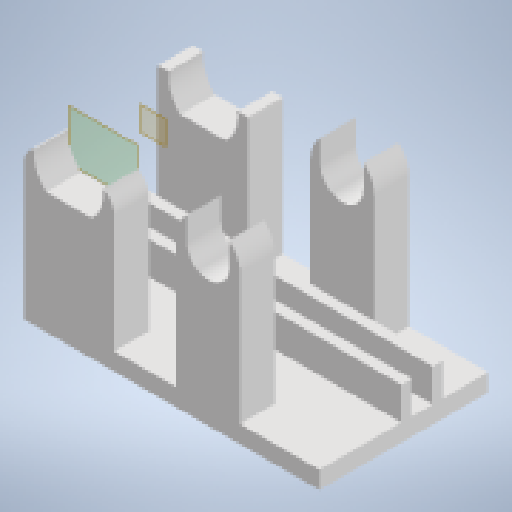
# Autodesk Inventor part: tempMotorHolder_V3
Saved by Autodesk Inventor 2023 (Build 270158000, 158)
## iProperties
Created: 2022-11-25
Part Number: tempMotorHolder_V3
Material: Generic
Document SubType Name: Modeling
Designer: shrey
Density: 1 g/cm^3
Appearance: Default
Author: shrey
Autodesk Inventor part; units mm, degrees
(part 1 of 2)
ref_plane "YZ Plane" through (0, 0, 0) normal (1, 0, 0) x (0, 1, 0)
ref_plane "XZ Plane" through (0, 0, 0) normal (0, 1, 0) x (-1, 0, 0)
ref_plane "XY Plane" through (0, 0, 0) normal (0, 0, 1) x (1, 0, 0)
ref_plane "Work Plane1" through (24.9677, 22.5561, 7.78) normal (0, 0, 1) x (1, 0, 0)
ref_plane "Work Plane2" through (24.8534, 22.5561, 22.06) normal (0, 0, -1) x (-1, 0, 0)
sketch "Sketch1" plane through (24.8534, 22.5561, 22.06) normal (0, 0, -1) x (-1, 0, 0)
  line L0 (6.3856, -7.5) -> (-6.6144, -7.5) construction
  line L1 (-6.6144, 7.5) -> (6.3856, 7.5) construction
  arc A0 (6.3856, -7.5) -> (6.3856, 7.5) centre (-0.2288, 0) ccw construction
  arc A1 (-6.6144, 7.5) -> (-6.6144, -7.5) centre (0, 0) ccw construction
  line L2 (6.4233, 7.6) -> (-6.6521, 7.6)
  arc A2 (-6.6521, 7.6) -> (-6.6521, -7.6) centre (0, 0) ccw
  line L3 (-6.6521, -7.6) -> (6.4233, -7.6)
  arc A3 (6.4233, -7.6) -> (6.4233, 7.6) centre (-0.2288, 0) ccw
  line L4 (9.7712, 0) -> (9.7712, 14.6932)
  line L5 (-10, 0) -> (-10, 14.6932)
  spline S0 degree 3 poles (-32.7358, 31.1377) (-32.7075, 31.029) (-32.6509, 30.8115) (-32.5759, 30.4828) (-32.5083, 30.1525) (-32.4494, 29.8206) (-32.3995, 29.4872) (-32.3592, 29.1525) (-32.3295, 28.8167) (-32.3114, 28.4801) (-32.307, 28.1991) (-32.3108, 27.9744) (-32.3179, 27.806) (-32.3291, 27.6378) (-32.3467, 27.4702) (-32.3629, 27.3307) (-32.3682, 27.2184) (-32.3676, 27.1341) (-32.3634, 27.0499) (-32.3544, 26.9661) (-32.3399, 26.883) (-32.3196, 26.8011) (-32.2931, 26.7211) (-32.2601, 26.6434) (-32.2203, 26.569) (-32.1734, 26.4988) (-32.12, 26.4335) (-32.0614, 26.3729) (-31.9958, 26.3197) (-31.9255, 26.2731) (-31.851, 26.2334) (-31.7455, 26.1941) (-31.611, 26.1536) (-31.4784, 26.1073) (-31.3701, 26.077) (-31.2864, 26.0653) (-31.2022, 26.0616) (-31.1178, 26.0661) (-31.0347, 26.0807) (-30.9532, 26.1021) (-30.874, 26.1312) (-30.798, 26.1681) (-30.7257, 26.2114) (-30.6571, 26.2606) (-30.5926, 26.3148) (-30.532, 26.3735) (-30.4754, 26.436) (-30.4225, 26.5017) (-30.3724, 26.5695) (-30.3107, 26.6634) (-30.2417, 26.7858) (-30.1574, 26.9317) (-30.0676, 27.0744) (-29.9742, 27.2147) (-29.8452, 27.3987) (-29.6764, 27.6233) (-29.4638, 27.8849) (-29.2422, 28.1391) (-29.0129, 28.3861) (-28.7764, 28.6264) (-28.5336, 28.8602) (-28.2847, 29.0876) (-28.0307, 29.3093) (-27.8571, 29.4519) (-27.7702, 29.5232) knots -1.078574 -1.078574 -1.078574 -1.078574 -1.044867 -1.011159 -0.977452 -0.943745 -0.910038 -0.876331 -0.842624 -0.808918 -0.775212 -0.758359 -0.741505 -0.724651 -0.707798 -0.690947 -0.68252 -0.674093 -0.665668 -0.657242 -0.648815 -0.640389 -0.631963 -0.623537 -0.61511 -0.606685 -0.598264 -0.589839 -0.581413 -0.57299 -0.564565 -0.556141 -0.539287 -0.522433 -0.514009 -0.505584 -0.49716 -0.488735 -0.48031 -0.471889 -0.463464 -0.455037 -0.446611 -0.438185 -0.429758 -0.421332 -0.412906 -0.40448 -0.396053 -0.387627 -0.370775 -0.353922 -0.337069 -0.320215 -0.303361 -0.269656 -0.235949 -0.202243 -0.168536 -0.134829 -0.101122 -0.067415 -0.033707 0 0 0 0 construction
  arc A4 (-26.4231, 28.9232) -> (-27.7702, 29.5232) centre (-40.1144, 0) ccw construction
  spline S1 degree 3 poles (-26.4231, 28.9232) (-26.4181, 28.8109) (-26.408, 28.5864) (-26.4029, 28.2493) (-26.4055, 27.9122) (-26.4168, 27.5753) (-26.4373, 27.2388) (-26.4676, 26.9031) (-26.5083, 26.5684) (-26.5606, 26.2354) (-26.6146, 25.9596) (-26.6651, 25.7407) (-26.707, 25.5774) (-26.753, 25.4152) (-26.8051, 25.2549) (-26.8499, 25.1218) (-26.8785, 25.0131) (-26.8954, 24.9305) (-26.9088, 24.8473) (-26.9174, 24.7634) (-26.9206, 24.6791) (-26.9177, 24.5948) (-26.9084, 24.511) (-26.8922, 24.4282) (-26.8688, 24.3471) (-26.8375, 24.2688) (-26.7989, 24.1938) (-26.7541, 24.1222) (-26.7011, 24.0566) (-26.642, 23.9964) (-26.5773, 23.9421) (-26.4823, 23.8817) (-26.3592, 23.8141) (-26.2391, 23.7413) (-26.1394, 23.6891) (-26.0601, 23.6603) (-25.9784, 23.6392) (-25.895, 23.626) (-25.8107, 23.623) (-25.7264, 23.627) (-25.6429, 23.639) (-25.561, 23.6592) (-25.4812, 23.6866) (-25.4039, 23.7204) (-25.3295, 23.7601) (-25.258, 23.8049) (-25.1897, 23.8543) (-25.1243, 23.9075) (-25.0612, 23.9634) (-24.9813, 24.0425) (-24.8884, 24.1479) (-24.7756, 24.2731) (-24.658, 24.3939) (-24.5376, 24.5118) (-24.3731, 24.6649) (-24.1613, 24.8495) (-23.8989, 25.0612) (-23.6294, 25.2637) (-23.3537, 25.4577) (-23.0724, 25.6436) (-22.7863, 25.8218) (-22.4955, 25.9924) (-22.201, 26.1565) (-22.0015, 26.2599) (-21.9018, 26.3116) knots -1.078574 -1.078574 -1.078574 -1.078574 -1.044867 -1.011159 -0.977452 -0.943745 -0.910038 -0.876331 -0.842624 -0.808918 -0.775212 -0.758359 -0.741505 -0.724651 -0.707798 -0.690947 -0.68252 -0.674093 -0.665668 -0.657242 -0.648815 -0.640389 -0.631963 -0.623537 -0.61511 -0.606685 -0.598264 -0.589839 -0.581413 -0.57299 -0.564565 -0.556141 -0.539287 -0.522433 -0.514009 -0.505584 -0.49716 -0.488735 -0.48031 -0.471889 -0.463464 -0.455037 -0.446611 -0.438185 -0.429758 -0.421332 -0.412906 -0.40448 -0.396053 -0.387627 -0.370775 -0.353922 -0.337069 -0.320215 -0.303361 -0.269656 -0.235949 -0.202243 -0.168536 -0.134829 -0.101122 -0.067415 -0.033707 0 0 0 0 construction
  arc A5 (-20.7088, 25.4446) -> (-21.9018, 26.3116) centre (-40.1144, 0) ccw construction
  spline S2 degree 3 poles (-20.7088, 25.4446) (-20.7272, 25.3337) (-20.764, 25.112) (-20.8292, 24.7812) (-20.9017, 24.4521) (-20.9829, 24.1249) (-21.0729, 23.8) (-21.1723, 23.4778) (-21.2818, 23.159) (-21.4021, 22.8441) (-21.5123, 22.5856) (-21.6073, 22.3819) (-21.6822, 22.2309) (-21.7608, 22.0818) (-21.8451, 21.9359) (-21.9167, 21.815) (-21.9672, 21.7146) (-22.0009, 21.6373) (-22.0313, 21.5587) (-22.0572, 21.4785) (-22.0778, 21.3967) (-22.0925, 21.3136) (-22.1008, 21.2297) (-22.1023, 21.1453) (-22.0962, 21.0612) (-22.0819, 20.978) (-22.0597, 20.8967) (-22.0308, 20.8174) (-21.9925, 20.7421) (-21.9472, 20.6709) (-21.8953, 20.6043) (-21.8149, 20.5256) (-21.7086, 20.4339) (-21.6063, 20.3377) (-21.5196, 20.2659) (-21.4479, 20.2212) (-21.3724, 20.1836) (-21.2936, 20.1533) (-21.2117, 20.1328) (-21.1285, 20.1193) (-21.0443, 20.1136) (-20.96, 20.1164) (-20.8762, 20.1266) (-20.7936, 20.1436) (-20.7125, 20.1669) (-20.6334, 20.1959) (-20.5562, 20.23) (-20.4812, 20.2685) (-20.4079, 20.31) (-20.3133, 20.3707) (-20.2005, 20.4545) (-20.0641, 20.5535) (-19.924, 20.6473) (-19.7817, 20.7375) (-19.589, 20.8531) (-19.3434, 20.9897) (-19.0427, 21.1422) (-18.737, 21.2842) (-18.427, 21.4166) (-18.1132, 21.54) (-17.7963, 21.6548) (-17.4764, 21.7613) (-17.1542, 21.8605) (-16.9376, 21.9202) (-16.8293, 21.95) knots -1.078574 -1.078574 -1.078574 -1.078574 -1.044867 -1.011159 -0.977452 -0.943745 -0.910038 -0.876331 -0.842624 -0.808918 -0.775212 -0.758359 -0.741505 -0.724651 -0.707798 -0.690947 -0.68252 -0.674093 -0.665668 -0.657242 -0.648815 -0.640389 -0.631963 -0.623537 -0.61511 -0.606685 -0.598264 -0.589839 -0.581413 -0.57299 -0.564565 -0.556141 -0.539287 -0.522433 -0.514009 -0.505584 -0.49716 -0.488735 -0.48031 -0.471889 -0.463464 -0.455037 -0.446611 -0.438185 -0.429758 -0.421332 -0.412906 -0.40448 -0.396053 -0.387627 -0.370775 -0.353922 -0.337069 -0.320215 -0.303361 -0.269656 -0.235949 -0.202243 -0.168536 -0.134829 -0.101122 -0.067415 -0.033707 0 0 0 0 construction
  arc A6 (-15.8427, 20.8539) -> (-16.8293, 21.95) centre (-40.1144, 0) ccw construction
  spline S3 degree 3 poles (-15.8427, 20.8539) (-15.8837, 20.7493) (-15.9658, 20.5401) (-16.0983, 20.2301) (-16.2377, 19.9232) (-16.3851, 19.62) (-16.5407, 19.3209) (-16.7049, 19.0265) (-16.8783, 18.7374) (-17.0615, 18.4544) (-17.223, 18.2245) (-17.3582, 18.045) (-17.4629, 17.9129) (-17.5708, 17.7834) (-17.6836, 17.6581) (-17.7787, 17.5548) (-17.8491, 17.4671) (-17.8981, 17.3985) (-17.9442, 17.3279) (-17.9862, 17.2548) (-18.0233, 17.1791) (-18.055, 17.1009) (-18.0806, 17.0205) (-18.0995, 16.9383) (-18.1111, 16.8547) (-18.1144, 16.7704) (-18.1096, 16.6862) (-18.0978, 16.6027) (-18.076, 16.5211) (-18.0465, 16.4421) (-18.0095, 16.3661) (-17.9473, 16.2724) (-17.8624, 16.1605) (-17.7823, 16.0452) (-17.7124, 15.957) (-17.6516, 15.8983) (-17.5856, 15.8458) (-17.5148, 15.7999) (-17.4389, 15.7628) (-17.3604, 15.7322) (-17.2792, 15.7092) (-17.1961, 15.6944) (-17.1121, 15.687) (-17.0277, 15.6864) (-16.9436, 15.6924) (-16.8601, 15.7042) (-16.7776, 15.7216) (-16.6962, 15.7436) (-16.6158, 15.769) (-16.5107, 15.8087) (-16.3829, 15.8672) (-16.2289, 15.9357) (-16.0724, 15.9983) (-15.9144, 16.0569) (-15.7019, 16.13) (-15.4333, 16.2125) (-15.1075, 16.2991) (-14.7789, 16.3745) (-14.4481, 16.4396) (-14.1156, 16.495) (-13.7817, 16.5414) (-13.4467, 16.579) (-13.1109, 16.6091) (-12.8866, 16.6224) (-12.7744, 16.6291) knots -1.078574 -1.078574 -1.078574 -1.078574 -1.044867 -1.011159 -0.977452 -0.943745 -0.910038 -0.876331 -0.842624 -0.808918 -0.775212 -0.758359 -0.741505 -0.724651 -0.707798 -0.690947 -0.68252 -0.674093 -0.665668 -0.657242 -0.648815 -0.640389 -0.631963 -0.623537 -0.61511 -0.606685 -0.598264 -0.589839 -0.581413 -0.57299 -0.564565 -0.556141 -0.539287 -0.522433 -0.514009 -0.505584 -0.49716 -0.488735 -0.48031 -0.471889 -0.463464 -0.455037 -0.446611 -0.438185 -0.429758 -0.421332 -0.412906 -0.40448 -0.396053 -0.387627 -0.370775 -0.353922 -0.337069 -0.320215 -0.303361 -0.269656 -0.235949 -0.202243 -0.168536 -0.134829 -0.101122 -0.067415 -0.033707 0 0 0 0 construction
  arc A7 (-12.0373, 15.3518) -> (-12.7744, 16.6291) centre (-40.1144, 0) ccw construction
  spline S4 degree 3 poles (-12.0373, 15.3518) (-12.0992, 15.258) (-12.223, 15.0705) (-12.417, 14.7948) (-12.6172, 14.5236) (-12.8245, 14.2577) (-13.0388, 13.9975) (-13.2606, 13.7437) (-13.4903, 13.4969) (-13.7283, 13.2581) (-13.9342, 13.0668) (-14.1037, 12.9194) (-14.2336, 12.8119) (-14.3661, 12.7077) (-14.5024, 12.6086) (-14.617, 12.5273) (-14.704, 12.4561) (-14.7662, 12.3993) (-14.826, 12.3398) (-14.8823, 12.277) (-14.9343, 12.2107) (-14.9816, 12.1408) (-15.0233, 12.0675) (-15.0589, 11.991) (-15.0876, 11.9117) (-15.1083, 11.8299) (-15.1212, 11.7465) (-15.127, 11.6624) (-15.1227, 11.578) (-15.1102, 11.4946) (-15.0899, 11.4126) (-15.0485, 11.308) (-14.9887, 11.1809) (-14.9343, 11.0514) (-14.8843, 10.9506) (-14.837, 10.8806) (-14.7834, 10.8156) (-14.7236, 10.7559) (-14.6572, 10.7039) (-14.5867, 10.6576) (-14.512, 10.6182) (-14.4339, 10.5864) (-14.3532, 10.5617) (-14.2708, 10.5436) (-14.1873, 10.532) (-14.1032, 10.5262) (-14.0188, 10.526) (-13.9347, 10.5306) (-13.8508, 10.5388) (-13.7397, 10.5558) (-13.6025, 10.5864) (-13.4377, 10.6214) (-13.2716, 10.6501) (-13.1048, 10.6746) (-12.8817, 10.7018) (-12.6019, 10.7267) (-12.2652, 10.7437) (-11.9281, 10.7491) (-11.591, 10.744) (-11.2542, 10.7291) (-10.918, 10.705) (-10.5825, 10.6722) (-10.2478, 10.6318) (-10.0256, 10.5982) (-9.9145, 10.5814) knots -1.078574 -1.078574 -1.078574 -1.078574 -1.044867 -1.011159 -0.977452 -0.943745 -0.910038 -0.876331 -0.842624 -0.808918 -0.775212 -0.758359 -0.741505 -0.724651 -0.707798 -0.690947 -0.68252 -0.674093 -0.665668 -0.657242 -0.648815 -0.640389 -0.631963 -0.623537 -0.61511 -0.606685 -0.598264 -0.589839 -0.581413 -0.57299 -0.564565 -0.556141 -0.539287 -0.522433 -0.514009 -0.505584 -0.49716 -0.488735 -0.48031 -0.471889 -0.463464 -0.455037 -0.446611 -0.438185 -0.429758 -0.421332 -0.412906 -0.40448 -0.396053 -0.387627 -0.370775 -0.353922 -0.337069 -0.320215 -0.303361 -0.269656 -0.235949 -0.202243 -0.168536 -0.134829 -0.101122 -0.067415 -0.033707 0 0 0 0 construction
  arc A8 (-9.459, 9.1788) -> (-9.9145, 10.5814) centre (-40.1144, 0) ccw construction
  spline S5 degree 3 poles (-9.459, 9.1788) (-9.5391, 9.0999) (-9.6991, 8.9422) (-9.9463, 8.7129) (-10.1985, 8.4892) (-10.4565, 8.2722) (-10.7202, 8.0623) (-10.99, 7.8601) (-11.266, 7.6665) (-11.5484, 7.4824) (-11.7895, 7.3381) (-11.986, 7.2291) (-12.1354, 7.151) (-12.2867, 7.0766) (-12.4406, 7.0081) (-12.5696, 6.9523) (-12.6695, 6.9008) (-12.7422, 6.8581) (-12.813, 6.8124) (-12.8811, 6.7627) (-12.9458, 6.7086) (-13.0066, 6.6501) (-13.0626, 6.5871) (-13.1134, 6.5197) (-13.158, 6.448) (-13.1952, 6.3723) (-13.2251, 6.2935) (-13.2483, 6.2123) (-13.2616, 6.129) (-13.2668, 6.0448) (-13.2639, 5.9604) (-13.2451, 5.8494) (-13.2131, 5.7127) (-13.1868, 5.5747) (-13.1589, 5.4657) (-13.1272, 5.3874) (-13.0882, 5.3126) (-13.0422, 5.2418) (-12.988, 5.1771) (-12.9287, 5.1172) (-12.8639, 5.0632) (-12.794, 5.0158) (-12.7203, 4.9749) (-12.6434, 4.9401) (-12.5641, 4.9113) (-12.483, 4.8882) (-12.4006, 4.8704) (-12.3173, 4.8574) (-12.2336, 4.848) (-12.1213, 4.8415) (-11.9809, 4.843) (-11.8123, 4.8429) (-11.6439, 4.8364) (-11.4757, 4.8257) (-11.2518, 4.806) (-10.9729, 4.7721) (-10.64, 4.7188) (-10.3092, 4.654) (-9.9805, 4.5789) (-9.6542, 4.4943) (-9.3303, 4.4008) (-9.0089, 4.299) (-8.69, 4.1899) (-8.4796, 4.1108) (-8.3744, 4.0713) knots -1.078574 -1.078574 -1.078574 -1.078574 -1.044867 -1.011159 -0.977452 -0.943745 -0.910038 -0.876331 -0.842624 -0.808918 -0.775212 -0.758359 -0.741505 -0.724651 -0.707798 -0.690947 -0.68252 -0.674093 -0.665668 -0.657242 -0.648815 -0.640389 -0.631963 -0.623537 -0.61511 -0.606685 -0.598264 -0.589839 -0.581413 -0.57299 -0.564565 -0.556141 -0.539287 -0.522433 -0.514009 -0.505584 -0.49716 -0.488735 -0.48031 -0.471889 -0.463464 -0.455037 -0.446611 -0.438185 -0.429758 -0.421332 -0.412906 -0.40448 -0.396053 -0.387627 -0.370775 -0.353922 -0.337069 -0.320215 -0.303361 -0.269656 -0.235949 -0.202243 -0.168536 -0.134829 -0.101122 -0.067415 -0.033707 0 0 0 0 construction
  arc A9 (-8.2206, 2.6046) -> (-8.3744, 4.0713) centre (-40.1144, 0) ccw construction
  spline S6 degree 3 poles (-8.2206, 2.6046) (-8.3152, 2.5441) (-8.5046, 2.4231) (-8.794, 2.2502) (-9.0872, 2.0839) (-9.3847, 1.9252) (-9.6863, 1.7747) (-9.9922, 1.6331) (-10.3024, 1.501) (-10.617, 1.3797) (-10.8828, 1.2887) (-11.0977, 1.2229) (-11.26, 1.1776) (-11.4235, 1.1363) (-11.5883, 1.1013) (-11.726, 1.0735) (-11.8345, 1.0439) (-11.9144, 1.0173) (-11.9932, 0.9873) (-12.0702, 0.9528) (-12.1447, 0.9134) (-12.2163, 0.8688) (-12.2842, 0.8188) (-12.3479, 0.7634) (-12.4064, 0.7026) (-12.4586, 0.6363) (-12.5042, 0.5653) (-12.5438, 0.4908) (-12.5741, 0.412) (-12.5967, 0.3307) (-12.6114, 0.2476) (-12.6161, 0.1352) (-12.6132, -0.0053) (-12.6162, -0.1457) (-12.6115, -0.2581) (-12.5968, -0.3413) (-12.5743, -0.4225) (-12.544, -0.5014) (-12.5044, -0.5759) (-12.4588, -0.6468) (-12.4067, -0.7132) (-12.3482, -0.774) (-12.2846, -0.8294) (-12.2166, -0.8794) (-12.1451, -0.9241) (-12.0705, -0.9635) (-11.9936, -0.998) (-11.9148, -1.028) (-11.8349, -1.0547) (-11.7265, -1.0844) (-11.5887, -1.1122) (-11.4239, -1.1473) (-11.2605, -1.1886) (-11.0982, -1.234) (-10.8833, -1.2999) (-10.6175, -1.391) (-10.303, -1.5124) (-9.9929, -1.6446) (-9.687, -1.7864) (-9.3854, -1.937) (-9.088, -2.0957) (-8.7949, -2.2622) (-8.5055, -2.4352) (-8.3162, -2.5563) (-8.2216, -2.6168) knots -1.078574 -1.078574 -1.078574 -1.078574 -1.044867 -1.011159 -0.977452 -0.943745 -0.910038 -0.876331 -0.842624 -0.808918 -0.775212 -0.758359 -0.741505 -0.724651 -0.707798 -0.690947 -0.68252 -0.674093 -0.665668 -0.657242 -0.648815 -0.640389 -0.631963 -0.623537 -0.61511 -0.606685 -0.598264 -0.589839 -0.581413 -0.57299 -0.564565 -0.556141 -0.539287 -0.522433 -0.514009 -0.505584 -0.49716 -0.488735 -0.48031 -0.471889 -0.463464 -0.455037 -0.446611 -0.438185 -0.429758 -0.421332 -0.412906 -0.40448 -0.396053 -0.387627 -0.370775 -0.353922 -0.337069 -0.320215 -0.303361 -0.269656 -0.235949 -0.202243 -0.168536 -0.134829 -0.101122 -0.067415 -0.033707 0 0 0 0 construction
  arc A10 (-8.376, -4.0834) -> (-8.2216, -2.6168) centre (-40.1144, 0) ccw construction
  spline S7 degree 3 poles (-8.376, -4.0834) (-8.4812, -4.1229) (-8.6916, -4.2019) (-9.0106, -4.3109) (-9.332, -4.4126) (-9.6559, -4.5059) (-9.9823, -4.5904) (-10.3109, -4.6654) (-10.6418, -4.73) (-10.9747, -4.7833) (-11.2536, -4.817) (-11.4775, -4.8367) (-11.6457, -4.8473) (-11.8142, -4.8537) (-11.9827, -4.8537) (-12.1232, -4.8522) (-12.2354, -4.8586) (-12.3192, -4.8681) (-12.4025, -4.881) (-12.4849, -4.8987) (-12.566, -4.9218) (-12.6453, -4.9506) (-12.7222, -4.9853) (-12.7959, -5.0263) (-12.8658, -5.0736) (-12.9306, -5.1276) (-12.99, -5.1875) (-13.0442, -5.2522) (-13.0903, -5.3229) (-13.1292, -5.3977) (-13.1609, -5.476) (-13.1889, -5.585) (-13.2152, -5.723) (-13.2474, -5.8597) (-13.2662, -5.9706) (-13.2691, -6.055) (-13.2639, -6.1392) (-13.2507, -6.2226) (-13.2275, -6.3037) (-13.1977, -6.3826) (-13.1604, -6.4584) (-13.1159, -6.53) (-13.0651, -6.5974) (-13.0091, -6.6605) (-12.9484, -6.719) (-12.8837, -6.7731) (-12.8156, -6.8228) (-12.7448, -6.8686) (-12.6722, -6.9113) (-12.5723, -6.9629) (-12.4433, -7.0187) (-12.2894, -7.0873) (-12.1381, -7.1617) (-11.9888, -7.2399) (-11.7923, -7.349) (-11.5513, -7.4933) (-11.2689, -7.6775) (-10.993, -7.8712) (-10.7233, -8.0735) (-10.4596, -8.2836) (-10.2017, -8.5007) (-9.9496, -8.7244) (-9.7026, -8.9538) (-9.5426, -9.1116) (-9.4625, -9.1905) knots -1.078574 -1.078574 -1.078574 -1.078574 -1.044867 -1.011159 -0.977452 -0.943745 -0.910038 -0.876331 -0.842624 -0.808918 -0.775212 -0.758359 -0.741505 -0.724651 -0.707798 -0.690947 -0.68252 -0.674093 -0.665668 -0.657242 -0.648815 -0.640389 -0.631963 -0.623537 -0.61511 -0.606685 -0.598264 -0.589839 -0.581413 -0.57299 -0.564565 -0.556141 -0.539287 -0.522433 -0.514009 -0.505584 -0.49716 -0.488735 -0.48031 -0.471889 -0.463464 -0.455037 -0.446611 -0.438185 -0.429758 -0.421332 -0.412906 -0.40448 -0.396053 -0.387627 -0.370775 -0.353922 -0.337069 -0.320215 -0.303361 -0.269656 -0.235949 -0.202243 -0.168536 -0.134829 -0.101122 -0.067415 -0.033707 0 0 0 0 construction
  arc A11 (-9.9185, -10.593) -> (-9.4625, -9.1905) centre (-40.1144, 0) ccw construction
  spline S8 degree 3 poles (-9.9185, -10.593) (-10.0296, -10.6097) (-10.2518, -10.6432) (-10.5866, -10.6835) (-10.9221, -10.7162) (-11.2583, -10.7401) (-11.5951, -10.7549) (-11.9322, -10.7599) (-12.2693, -10.7543) (-12.606, -10.7372) (-12.8858, -10.7123) (-13.1089, -10.6849) (-13.2756, -10.6603) (-13.4417, -10.6316) (-13.6066, -10.5966) (-13.7437, -10.5659) (-13.8548, -10.5488) (-13.9387, -10.5406) (-14.0229, -10.536) (-14.1072, -10.5362) (-14.1913, -10.5419) (-14.2749, -10.5535) (-14.3573, -10.5716) (-14.4379, -10.5963) (-14.5161, -10.628) (-14.5908, -10.6674) (-14.6613, -10.7136) (-14.7278, -10.7656) (-14.7875, -10.8252) (-14.8412, -10.8903) (-14.8885, -10.9603) (-14.9385, -11.0611) (-14.9929, -11.1905) (-15.0528, -11.3176) (-15.0942, -11.4222) (-15.1146, -11.5042) (-15.1271, -11.5876) (-15.1315, -11.6719) (-15.1257, -11.7561) (-15.1129, -11.8394) (-15.0922, -11.9213) (-15.0635, -12.0006) (-15.0279, -12.0771) (-14.9862, -12.1504) (-14.939, -12.2203) (-14.887, -12.2867) (-14.8307, -12.3495) (-14.771, -12.4089) (-14.7088, -12.4658) (-14.6218, -12.537) (-14.5073, -12.6184) (-14.371, -12.7175) (-14.2385, -12.8218) (-14.1087, -12.9293) (-13.9392, -13.0769) (-13.7334, -13.2682) (-13.4955, -13.5071) (-13.2659, -13.7539) (-13.0442, -14.0078) (-12.8299, -14.2681) (-12.6228, -14.5341) (-12.4227, -14.8054) (-12.2287, -15.0811) (-12.105, -15.2687) (-12.0432, -15.3625) knots -1.078574 -1.078574 -1.078574 -1.078574 -1.044867 -1.011159 -0.977452 -0.943745 -0.910038 -0.876331 -0.842624 -0.808918 -0.775212 -0.758359 -0.741505 -0.724651 -0.707798 -0.690947 -0.68252 -0.674093 -0.665668 -0.657242 -0.648815 -0.640389 -0.631963 -0.623537 -0.61511 -0.606685 -0.598264 -0.589839 -0.581413 -0.57299 -0.564565 -0.556141 -0.539287 -0.522433 -0.514009 -0.505584 -0.49716 -0.488735 -0.48031 -0.471889 -0.463464 -0.455037 -0.446611 -0.438185 -0.429758 -0.421332 -0.412906 -0.40448 -0.396053 -0.387627 -0.370775 -0.353922 -0.337069 -0.320215 -0.303361 -0.269656 -0.235949 -0.202243 -0.168536 -0.134829 -0.101122 -0.067415 -0.033707 0 0 0 0 construction
  arc A12 (-12.7808, -16.6395) -> (-12.0432, -15.3625) centre (-40.1144, 0) ccw construction
  spline S9 degree 3 poles (-12.7808, -16.6395) (-12.8929, -16.6328) (-13.1173, -16.6194) (-13.453, -16.5892) (-13.788, -16.5514) (-14.1219, -16.5049) (-14.4544, -16.4494) (-14.7852, -16.3842) (-15.1137, -16.3087) (-15.4395, -16.2219) (-15.7081, -16.1393) (-15.9206, -16.0662) (-16.0785, -16.0075) (-16.235, -15.9448) (-16.389, -15.8763) (-16.5167, -15.8177) (-16.6219, -15.778) (-16.7022, -15.7525) (-16.7836, -15.7305) (-16.8661, -15.7131) (-16.9496, -15.7012) (-17.0337, -15.6952) (-17.1181, -15.6957) (-17.2021, -15.7031) (-17.2852, -15.7179) (-17.3664, -15.7409) (-17.445, -15.7715) (-17.5208, -15.8085) (-17.5917, -15.8544) (-17.6577, -15.9069) (-17.7185, -15.9655) (-17.7884, -16.0537) (-17.8685, -16.169) (-17.9535, -16.2809) (-18.0158, -16.3746) (-18.0528, -16.4505) (-18.0823, -16.5295) (-18.1041, -16.6111) (-18.116, -16.6946) (-18.1208, -16.7788) (-18.1176, -16.8632) (-18.106, -16.9467) (-18.0871, -17.029) (-18.0615, -17.1094) (-18.0299, -17.1875) (-17.9928, -17.2633) (-17.9508, -17.3364) (-17.9047, -17.407) (-17.8557, -17.4756) (-17.7854, -17.5633) (-17.6904, -17.6667) (-17.5776, -17.792) (-17.4697, -17.9215) (-17.3651, -18.0537) (-17.23, -18.2332) (-17.0685, -18.4632) (-16.8855, -18.7463) (-16.7122, -19.0355) (-16.5481, -19.33) (-16.3926, -19.6291) (-16.2453, -19.9323) (-16.106, -20.2393) (-15.9737, -20.5493) (-15.8917, -20.7586) (-15.8507, -20.8632) knots -1.078574 -1.078574 -1.078574 -1.078574 -1.044867 -1.011159 -0.977452 -0.943745 -0.910038 -0.876331 -0.842624 -0.808918 -0.775212 -0.758359 -0.741505 -0.724651 -0.707798 -0.690947 -0.68252 -0.674093 -0.665668 -0.657242 -0.648815 -0.640389 -0.631963 -0.623537 -0.61511 -0.606685 -0.598264 -0.589839 -0.581413 -0.57299 -0.564565 -0.556141 -0.539287 -0.522433 -0.514009 -0.505584 -0.49716 -0.488735 -0.48031 -0.471889 -0.463464 -0.455037 -0.446611 -0.438185 -0.429758 -0.421332 -0.412906 -0.40448 -0.396053 -0.387627 -0.370775 -0.353922 -0.337069 -0.320215 -0.303361 -0.269656 -0.235949 -0.202243 -0.168536 -0.134829 -0.101122 -0.067415 -0.033707 0 0 0 0 construction
  arc A13 (-16.8376, -21.9589) -> (-15.8507, -20.8632) centre (-40.1144, 0) ccw construction
  spline S10 degree 3 poles (-16.8376, -21.9589) (-16.946, -21.929) (-17.1626, -21.8693) (-17.4847, -21.7699) (-17.8045, -21.6633) (-18.1215, -21.5484) (-18.4352, -21.4249) (-18.7451, -21.2924) (-19.0508, -21.1502) (-19.3514, -20.9976) (-19.5969, -20.861) (-19.7896, -20.7453) (-19.9319, -20.655) (-20.072, -20.5612) (-20.2083, -20.4621) (-20.3211, -20.3783) (-20.4157, -20.3175) (-20.489, -20.276) (-20.564, -20.2375) (-20.6411, -20.2034) (-20.7203, -20.1743) (-20.8013, -20.151) (-20.8839, -20.134) (-20.9677, -20.1237) (-21.052, -20.1209) (-21.1362, -20.1265) (-21.2194, -20.1401) (-21.3013, -20.1605) (-21.3802, -20.1907) (-21.4557, -20.2283) (-21.5273, -20.273) (-21.614, -20.3447) (-21.7164, -20.4409) (-21.8228, -20.5326) (-21.9032, -20.6113) (-21.9551, -20.6779) (-22.0005, -20.749) (-22.0388, -20.8243) (-22.0677, -20.9036) (-22.0899, -20.9849) (-22.1043, -21.0681) (-22.1104, -21.1522) (-22.109, -21.2366) (-22.1007, -21.3205) (-22.086, -21.4036) (-22.0654, -21.4854) (-22.0396, -21.5656) (-22.0092, -21.6442) (-21.9755, -21.7215) (-21.925, -21.8219) (-21.8535, -21.9429) (-21.7693, -22.0889) (-21.6907, -22.238) (-21.6158, -22.389) (-21.521, -22.5927) (-21.4108, -22.8512) (-21.2906, -23.1662) (-21.1813, -23.4851) (-21.082, -23.8073) (-20.9921, -24.1322) (-20.9111, -24.4594) (-20.8386, -24.7886) (-20.7736, -25.1194) (-20.7369, -25.3411) (-20.7186, -25.452) knots -1.078574 -1.078574 -1.078574 -1.078574 -1.044867 -1.011159 -0.977452 -0.943745 -0.910038 -0.876331 -0.842624 -0.808918 -0.775212 -0.758359 -0.741505 -0.724651 -0.707798 -0.690947 -0.68252 -0.674093 -0.665668 -0.657242 -0.648815 -0.640389 -0.631963 -0.623537 -0.61511 -0.606685 -0.598264 -0.589839 -0.581413 -0.57299 -0.564565 -0.556141 -0.539287 -0.522433 -0.514009 -0.505584 -0.49716 -0.488735 -0.48031 -0.471889 -0.463464 -0.455037 -0.446611 -0.438185 -0.429758 -0.421332 -0.412906 -0.40448 -0.396053 -0.387627 -0.370775 -0.353922 -0.337069 -0.320215 -0.303361 -0.269656 -0.235949 -0.202243 -0.168536 -0.134829 -0.101122 -0.067415 -0.033707 0 0 0 0 construction
  arc A14 (-21.9118, -26.3186) -> (-20.7186, -25.452) centre (-40.1144, 0) ccw construction
  spline S11 degree 3 poles (-21.9118, -26.3186) (-22.0115, -26.2668) (-22.211, -26.1633) (-22.5055, -25.9992) (-22.7961, -25.8284) (-23.0822, -25.6501) (-23.3634, -25.4641) (-23.639, -25.27) (-23.9085, -25.0674) (-24.1708, -24.8556) (-24.3825, -24.6709) (-24.5469, -24.5177) (-24.6674, -24.3998) (-24.7849, -24.2789) (-24.8976, -24.1537) (-24.9905, -24.0483) (-25.0704, -23.9691) (-25.1334, -23.9132) (-25.1988, -23.86) (-25.2671, -23.8106) (-25.3385, -23.7657) (-25.413, -23.7261) (-25.4902, -23.6922) (-25.57, -23.6648) (-25.6519, -23.6445) (-25.7355, -23.6325) (-25.8197, -23.6284) (-25.904, -23.6314) (-25.9874, -23.6446) (-26.0691, -23.6656) (-26.1485, -23.6945) (-26.2482, -23.7466) (-26.3683, -23.8194) (-26.4914, -23.887) (-26.5865, -23.9472) (-26.6511, -24.0015) (-26.7103, -24.0617) (-26.7634, -24.1273) (-26.8081, -24.1989) (-26.8468, -24.2738) (-26.8782, -24.3522) (-26.9016, -24.4332) (-26.9178, -24.516) (-26.9271, -24.5999) (-26.93, -24.6842) (-26.9269, -24.7684) (-26.9183, -24.8523) (-26.9049, -24.9355) (-26.8881, -25.0181) (-26.8595, -25.1269) (-26.8147, -25.26) (-26.7627, -25.4203) (-26.7168, -25.5825) (-26.675, -25.7458) (-26.6246, -25.9648) (-26.5706, -26.2405) (-26.5185, -26.5736) (-26.4779, -26.9083) (-26.4477, -27.2441) (-26.4274, -27.5806) (-26.4161, -27.9175) (-26.4137, -28.2546) (-26.4189, -28.5917) (-26.4291, -28.8161) (-26.4342, -28.9284) knots -1.078574 -1.078574 -1.078574 -1.078574 -1.044867 -1.011159 -0.977452 -0.943745 -0.910038 -0.876331 -0.842624 -0.808918 -0.775212 -0.758359 -0.741505 -0.724651 -0.707798 -0.690947 -0.68252 -0.674093 -0.665668 -0.657242 -0.648815 -0.640389 -0.631963 -0.623537 -0.61511 -0.606685 -0.598264 -0.589839 -0.581413 -0.57299 -0.564565 -0.556141 -0.539287 -0.522433 -0.514009 -0.505584 -0.49716 -0.488735 -0.48031 -0.471889 -0.463464 -0.455037 -0.446611 -0.438185 -0.429758 -0.421332 -0.412906 -0.40448 -0.396053 -0.387627 -0.370775 -0.353922 -0.337069 -0.320215 -0.303361 -0.269656 -0.235949 -0.202243 -0.168536 -0.134829 -0.101122 -0.067415 -0.033707 0 0 0 0 construction
  arc A15 (-27.7815, -29.528) -> (-26.4342, -28.9284) centre (-40.1144, 0) ccw construction
  spline S12 degree 3 poles (-27.7815, -29.528) (-27.8683, -29.4566) (-28.0419, -29.3139) (-28.2958, -29.0921) (-28.5446, -28.8647) (-28.7874, -28.6308) (-29.0237, -28.3904) (-29.253, -28.1432) (-29.4744, -27.889) (-29.687, -27.6273) (-29.8557, -27.4026) (-29.9846, -27.2186) (-30.0779, -27.0782) (-30.1677, -26.9355) (-30.252, -26.7896) (-30.3209, -26.6672) (-30.3826, -26.5732) (-30.4327, -26.5054) (-30.4855, -26.4397) (-30.5421, -26.3772) (-30.6026, -26.3185) (-30.6672, -26.2642) (-30.7357, -26.215) (-30.808, -26.1716) (-30.8839, -26.1347) (-30.9631, -26.1056) (-31.0447, -26.0841) (-31.1278, -26.0695) (-31.2121, -26.065) (-31.2964, -26.0687) (-31.38, -26.0804) (-31.4884, -26.1106) (-31.621, -26.1568) (-31.7555, -26.1973) (-31.861, -26.2365) (-31.9355, -26.2762) (-32.0059, -26.3228) (-32.0715, -26.3759) (-32.1301, -26.4366) (-32.1835, -26.5019) (-32.2305, -26.572) (-32.2703, -26.6464) (-32.3033, -26.724) (-32.3299, -26.8041) (-32.3502, -26.8859) (-32.3647, -26.969) (-32.3738, -27.0528) (-32.378, -27.137) (-32.3786, -27.2213) (-32.3733, -27.3336) (-32.3572, -27.4732) (-32.3396, -27.6408) (-32.3285, -27.809) (-32.3215, -27.9774) (-32.3177, -28.2021) (-32.3223, -28.483) (-32.3406, -28.8197) (-32.3704, -29.1555) (-32.4107, -29.4902) (-32.4608, -29.8235) (-32.5198, -30.1554) (-32.5876, -30.4857) (-32.6627, -30.8143) (-32.7194, -31.0318) (-32.7477, -31.1405) knots -1.078574 -1.078574 -1.078574 -1.078574 -1.044867 -1.011159 -0.977452 -0.943745 -0.910038 -0.876331 -0.842624 -0.808918 -0.775212 -0.758359 -0.741505 -0.724651 -0.707798 -0.690947 -0.68252 -0.674093 -0.665668 -0.657242 -0.648815 -0.640389 -0.631963 -0.623537 -0.61511 -0.606685 -0.598264 -0.589839 -0.581413 -0.57299 -0.564565 -0.556141 -0.539287 -0.522433 -0.514009 -0.505584 -0.49716 -0.488735 -0.48031 -0.471889 -0.463464 -0.455037 -0.446611 -0.438185 -0.429758 -0.421332 -0.412906 -0.40448 -0.396053 -0.387627 -0.370775 -0.353922 -0.337069 -0.320215 -0.303361 -0.269656 -0.235949 -0.202243 -0.168536 -0.134829 -0.101122 -0.067415 -0.033707 0 0 0 0 construction
  arc A16 (-34.1902, -31.4469) -> (-32.7477, -31.1405) centre (-40.1144, 0) ccw construction
  spline S13 degree 3 poles (-34.1902, -31.4469) (-34.2603, -31.359) (-34.4004, -31.1833) (-34.6027, -30.9136) (-34.7987, -30.6394) (-34.9876, -30.3601) (-35.1688, -30.0759) (-35.3416, -29.7864) (-35.5054, -29.4917) (-35.6589, -29.1916) (-35.7772, -28.9367) (-35.8651, -28.7299) (-35.9271, -28.5732) (-35.9853, -28.415) (-36.0374, -28.2547) (-36.0793, -28.1206) (-36.1201, -28.0159) (-36.155, -27.9391) (-36.1931, -27.8639) (-36.2354, -27.791) (-36.2824, -27.721) (-36.3342, -27.6544) (-36.3911, -27.5921) (-36.4528, -27.5346) (-36.5194, -27.4828) (-36.5908, -27.4378) (-36.6661, -27.3998) (-36.7443, -27.3683) (-36.8259, -27.3463) (-36.9091, -27.3324) (-36.9933, -27.3264) (-37.1056, -27.3335) (-37.2449, -27.3511) (-37.3849, -27.3628) (-37.4962, -27.3792) (-37.5774, -27.4025) (-37.6559, -27.4334) (-37.7311, -27.4718) (-37.8011, -27.5189) (-37.8669, -27.5717) (-37.9274, -27.6305) (-37.9818, -27.695) (-38.0302, -27.7641) (-38.0729, -27.8368) (-38.1098, -27.9127) (-38.1412, -27.9909) (-38.1675, -28.071) (-38.1891, -28.1525) (-38.2073, -28.2348) (-38.2255, -28.3458) (-38.2387, -28.4856) (-38.2564, -28.6532) (-38.2804, -28.8201) (-38.3086, -28.9863) (-38.3517, -29.2068) (-38.4145, -29.4807) (-38.5024, -29.8062) (-38.6014, -30.1284) (-38.7104, -30.4474) (-38.8287, -30.7631) (-38.9555, -31.0755) (-39.0904, -31.3844) (-39.2322, -31.6902) (-39.3328, -31.8912) (-39.3831, -31.9916) knots -1.078574 -1.078574 -1.078574 -1.078574 -1.044867 -1.011159 -0.977452 -0.943745 -0.910038 -0.876331 -0.842624 -0.808918 -0.775212 -0.758359 -0.741505 -0.724651 -0.707798 -0.690947 -0.68252 -0.674093 -0.665668 -0.657242 -0.648815 -0.640389 -0.631963 -0.623537 -0.61511 -0.606685 -0.598264 -0.589839 -0.581413 -0.57299 -0.564565 -0.556141 -0.539287 -0.522433 -0.514009 -0.505584 -0.49716 -0.488735 -0.48031 -0.471889 -0.463464 -0.455037 -0.446611 -0.438185 -0.429758 -0.421332 -0.412906 -0.40448 -0.396053 -0.387627 -0.370775 -0.353922 -0.337069 -0.320215 -0.303361 -0.269656 -0.235949 -0.202243 -0.168536 -0.134829 -0.101122 -0.067415 -0.033707 0 0 0 0 construction
  arc A17 (-40.8579, -31.9914) -> (-39.3831, -31.9916) centre (-40.1144, 0) ccw construction
  spline S14 degree 3 poles (-40.8579, -31.9914) (-40.9081, -31.8909) (-41.0087, -31.6899) (-41.1504, -31.384) (-41.2852, -31.075) (-41.4118, -30.7626) (-41.53, -30.4469) (-41.6389, -30.1278) (-41.7378, -29.8055) (-41.8255, -29.48) (-41.8883, -29.2061) (-41.9312, -28.9856) (-41.9593, -28.8194) (-41.9833, -28.6525) (-42.0009, -28.4849) (-42.0141, -28.345) (-42.0322, -28.2341) (-42.0504, -28.1518) (-42.072, -28.0703) (-42.0982, -27.9902) (-42.1296, -27.9119) (-42.1665, -27.8361) (-42.2091, -27.7633) (-42.2576, -27.6942) (-42.3119, -27.6296) (-42.3724, -27.5708) (-42.4382, -27.518) (-42.5082, -27.4709) (-42.5834, -27.4325) (-42.6618, -27.4015) (-42.743, -27.3782) (-42.8543, -27.3617) (-42.9943, -27.35) (-43.1336, -27.3323) (-43.2459, -27.3252) (-43.3301, -27.3311) (-43.4133, -27.3451) (-43.4949, -27.367) (-43.5731, -27.3985) (-43.6485, -27.4364) (-43.7199, -27.4814) (-43.7865, -27.5332) (-43.8483, -27.5907) (-43.9051, -27.653) (-43.957, -27.7195) (-44.004, -27.7895) (-44.0464, -27.8624) (-44.0844, -27.9376) (-44.1193, -28.0143) (-44.1602, -28.1191) (-44.2022, -28.2531) (-44.2543, -28.4134) (-44.3125, -28.5716) (-44.3747, -28.7283) (-44.4626, -28.9351) (-44.581, -29.1899) (-44.7347, -29.49) (-44.8985, -29.7846) (-45.0715, -30.074) (-45.2528, -30.3582) (-45.4417, -30.6373) (-45.6379, -30.9115) (-45.8402, -31.1811) (-45.9804, -31.3568) (-46.0505, -31.4446) knots -1.078574 -1.078574 -1.078574 -1.078574 -1.044867 -1.011159 -0.977452 -0.943745 -0.910038 -0.876331 -0.842624 -0.808918 -0.775212 -0.758359 -0.741505 -0.724651 -0.707798 -0.690947 -0.68252 -0.674093 -0.665668 -0.657242 -0.648815 -0.640389 -0.631963 -0.623537 -0.61511 -0.606685 -0.598264 -0.589839 -0.581413 -0.57299 -0.564565 -0.556141 -0.539287 -0.522433 -0.514009 -0.505584 -0.49716 -0.488735 -0.48031 -0.471889 -0.463464 -0.455037 -0.446611 -0.438185 -0.429758 -0.421332 -0.412906 -0.40448 -0.396053 -0.387627 -0.370775 -0.353922 -0.337069 -0.320215 -0.303361 -0.269656 -0.235949 -0.202243 -0.168536 -0.134829 -0.101122 -0.067415 -0.033707 0 0 0 0 construction
  arc A18 (-47.493, -31.1377) -> (-46.0505, -31.4446) centre (-40.1144, 0) ccw construction
  spline S15 degree 3 poles (-47.493, -31.1377) (-47.5213, -31.029) (-47.5778, -30.8115) (-47.6529, -30.4828) (-47.7204, -30.1525) (-47.7794, -29.8206) (-47.8293, -29.4872) (-47.8695, -29.1525) (-47.8992, -28.8167) (-47.9174, -28.4801) (-47.9218, -28.1991) (-47.9179, -27.9744) (-47.9109, -27.806) (-47.8997, -27.6378) (-47.8821, -27.4702) (-47.8659, -27.3307) (-47.8605, -27.2184) (-47.8612, -27.1341) (-47.8653, -27.0499) (-47.8743, -26.9661) (-47.8888, -26.883) (-47.9091, -26.8011) (-47.9357, -26.7211) (-47.9687, -26.6434) (-48.0084, -26.569) (-48.0554, -26.4988) (-48.1087, -26.4335) (-48.1674, -26.3729) (-48.2329, -26.3197) (-48.3033, -26.2731) (-48.3778, -26.2334) (-48.4833, -26.1941) (-48.6177, -26.1536) (-48.7503, -26.1073) (-48.8587, -26.077) (-48.9423, -26.0653) (-49.0266, -26.0616) (-49.1109, -26.0661) (-49.194, -26.0807) (-49.2756, -26.1021) (-49.3548, -26.1312) (-49.4307, -26.1681) (-49.5031, -26.2114) (-49.5716, -26.2606) (-49.6362, -26.3148) (-49.6968, -26.3735) (-49.7533, -26.436) (-49.8062, -26.5017) (-49.8563, -26.5695) (-49.918, -26.6634) (-49.987, -26.7858) (-50.0713, -26.9317) (-50.1612, -27.0744) (-50.2545, -27.2147) (-50.3835, -27.3987) (-50.5523, -27.6233) (-50.765, -27.8849) (-50.9865, -28.1391) (-51.2159, -28.3861) (-51.4523, -28.6264) (-51.6952, -28.8602) (-51.9441, -29.0876) (-52.198, -29.3093) (-52.3717, -29.4519) (-52.4585, -29.5232) knots -1.078574 -1.078574 -1.078574 -1.078574 -1.044867 -1.011159 -0.977452 -0.943745 -0.910038 -0.876331 -0.842624 -0.808918 -0.775212 -0.758359 -0.741505 -0.724651 -0.707798 -0.690947 -0.68252 -0.674093 -0.665668 -0.657242 -0.648815 -0.640389 -0.631963 -0.623537 -0.61511 -0.606685 -0.598264 -0.589839 -0.581413 -0.57299 -0.564565 -0.556141 -0.539287 -0.522433 -0.514009 -0.505584 -0.49716 -0.488735 -0.48031 -0.471889 -0.463464 -0.455037 -0.446611 -0.438185 -0.429758 -0.421332 -0.412906 -0.40448 -0.396053 -0.387627 -0.370775 -0.353922 -0.337069 -0.320215 -0.303361 -0.269656 -0.235949 -0.202243 -0.168536 -0.134829 -0.101122 -0.067415 -0.033707 0 0 0 0 construction
  arc A19 (-53.8056, -28.9232) -> (-52.4585, -29.5232) centre (-40.1144, 0) ccw construction
  spline S16 degree 3 poles (-53.8056, -28.9232) (-53.8107, -28.8109) (-53.8208, -28.5864) (-53.8259, -28.2493) (-53.8233, -27.9122) (-53.8119, -27.5753) (-53.7915, -27.2388) (-53.7612, -26.9031) (-53.7204, -26.5684) (-53.6682, -26.2354) (-53.6141, -25.9596) (-53.5636, -25.7407) (-53.5217, -25.5774) (-53.4758, -25.4152) (-53.4237, -25.2549) (-53.3788, -25.1218) (-53.3503, -25.0131) (-53.3334, -24.9305) (-53.32, -24.8473) (-53.3113, -24.7634) (-53.3082, -24.6791) (-53.3111, -24.5948) (-53.3204, -24.511) (-53.3365, -24.4282) (-53.3599, -24.3471) (-53.3913, -24.2688) (-53.4299, -24.1938) (-53.4746, -24.1222) (-53.5277, -24.0566) (-53.5868, -23.9964) (-53.6515, -23.9421) (-53.7464, -23.8817) (-53.8695, -23.8141) (-53.9896, -23.7413) (-54.0893, -23.6891) (-54.1687, -23.6603) (-54.2504, -23.6392) (-54.3338, -23.626) (-54.4181, -23.623) (-54.5023, -23.627) (-54.5859, -23.639) (-54.6678, -23.6592) (-54.7476, -23.6866) (-54.8249, -23.7204) (-54.8993, -23.7601) (-54.9707, -23.8049) (-55.0391, -23.8543) (-55.1045, -23.9075) (-55.1675, -23.9634) (-55.2474, -24.0425) (-55.3404, -24.1479) (-55.4532, -24.2731) (-55.5707, -24.3939) (-55.6912, -24.5118) (-55.8557, -24.6649) (-56.0675, -24.8495) (-56.3299, -25.0612) (-56.5994, -25.2637) (-56.8751, -25.4577) (-57.1563, -25.6436) (-57.4425, -25.8218) (-57.7332, -25.9924) (-58.0277, -26.1565) (-58.2272, -26.2599) (-58.327, -26.3116) knots -1.078574 -1.078574 -1.078574 -1.078574 -1.044867 -1.011159 -0.977452 -0.943745 -0.910038 -0.876331 -0.842624 -0.808918 -0.775212 -0.758359 -0.741505 -0.724651 -0.707798 -0.690947 -0.68252 -0.674093 -0.665668 -0.657242 -0.648815 -0.640389 -0.631963 -0.623537 -0.61511 -0.606685 -0.598264 -0.589839 -0.581413 -0.57299 -0.564565 -0.556141 -0.539287 -0.522433 -0.514009 -0.505584 -0.49716 -0.488735 -0.48031 -0.471889 -0.463464 -0.455037 -0.446611 -0.438185 -0.429758 -0.421332 -0.412906 -0.40448 -0.396053 -0.387627 -0.370775 -0.353922 -0.337069 -0.320215 -0.303361 -0.269656 -0.235949 -0.202243 -0.168536 -0.134829 -0.101122 -0.067415 -0.033707 0 0 0 0 construction
  arc A20 (-59.5199, -25.4446) -> (-58.327, -26.3116) centre (-40.1144, 0) ccw construction
  spline S17 degree 3 poles (-59.5199, -25.4446) (-59.5015, -25.3337) (-59.4647, -25.112) (-59.3996, -24.7812) (-59.327, -24.4521) (-59.2458, -24.1249) (-59.1558, -23.8) (-59.0564, -23.4778) (-58.947, -23.159) (-58.8267, -22.8441) (-58.7164, -22.5856) (-58.6215, -22.3819) (-58.5466, -22.2309) (-58.4679, -22.0818) (-58.3837, -21.9359) (-58.3121, -21.815) (-58.2615, -21.7146) (-58.2278, -21.6373) (-58.1974, -21.5587) (-58.1715, -21.4785) (-58.151, -21.3967) (-58.1362, -21.3136) (-58.1279, -21.2297) (-58.1265, -21.1453) (-58.1325, -21.0612) (-58.1469, -20.978) (-58.1691, -20.8967) (-58.198, -20.8174) (-58.2362, -20.7421) (-58.2815, -20.6709) (-58.3335, -20.6043) (-58.4138, -20.5256) (-58.5202, -20.4339) (-58.6225, -20.3377) (-58.7092, -20.2659) (-58.7808, -20.2212) (-58.8563, -20.1836) (-58.9352, -20.1533) (-59.017, -20.1328) (-59.1003, -20.1193) (-59.1845, -20.1136) (-59.2688, -20.1164) (-59.3525, -20.1266) (-59.4352, -20.1436) (-59.5162, -20.1669) (-59.5954, -20.1959) (-59.6725, -20.23) (-59.7475, -20.2685) (-59.8209, -20.31) (-59.9155, -20.3707) (-60.0283, -20.4545) (-60.1646, -20.5535) (-60.3047, -20.6473) (-60.4471, -20.7375) (-60.6398, -20.8531) (-60.8853, -20.9897) (-61.186, -21.1422) (-61.4918, -21.2842) (-61.8018, -21.4166) (-62.1155, -21.54) (-62.4325, -21.6548) (-62.7523, -21.7613) (-63.0745, -21.8605) (-63.2912, -21.9202) (-63.3995, -21.95) knots -1.078574 -1.078574 -1.078574 -1.078574 -1.044867 -1.011159 -0.977452 -0.943745 -0.910038 -0.876331 -0.842624 -0.808918 -0.775212 -0.758359 -0.741505 -0.724651 -0.707798 -0.690947 -0.68252 -0.674093 -0.665668 -0.657242 -0.648815 -0.640389 -0.631963 -0.623537 -0.61511 -0.606685 -0.598264 -0.589839 -0.581413 -0.57299 -0.564565 -0.556141 -0.539287 -0.522433 -0.514009 -0.505584 -0.49716 -0.488735 -0.48031 -0.471889 -0.463464 -0.455037 -0.446611 -0.438185 -0.429758 -0.421332 -0.412906 -0.40448 -0.396053 -0.387627 -0.370775 -0.353922 -0.337069 -0.320215 -0.303361 -0.269656 -0.235949 -0.202243 -0.168536 -0.134829 -0.101122 -0.067415 -0.033707 0 0 0 0 construction
  arc A21 (-64.3861, -20.8539) -> (-63.3995, -21.95) centre (-40.1144, 0) ccw construction
  spline S18 degree 3 poles (-64.3861, -20.8539) (-64.345, -20.7493) (-64.263, -20.5401) (-64.1305, -20.2301) (-63.991, -19.9232) (-63.8436, -19.62) (-63.688, -19.3209) (-63.5238, -19.0265) (-63.3505, -18.7374) (-63.1673, -18.4544) (-63.0057, -18.2245) (-62.8705, -18.045) (-62.7659, -17.9129) (-62.6579, -17.7834) (-62.5452, -17.6581) (-62.45, -17.5548) (-62.3797, -17.4671) (-62.3307, -17.3985) (-62.2846, -17.3279) (-62.2426, -17.2548) (-62.2054, -17.1791) (-62.1738, -17.1009) (-62.1482, -17.0205) (-62.1292, -16.9383) (-62.1176, -16.8547) (-62.1144, -16.7704) (-62.1192, -16.6862) (-62.131, -16.6027) (-62.1527, -16.5211) (-62.1822, -16.4421) (-62.2192, -16.3661) (-62.2815, -16.2724) (-62.3664, -16.1605) (-62.4465, -16.0452) (-62.5164, -15.957) (-62.5771, -15.8983) (-62.6432, -15.8458) (-62.714, -15.7999) (-62.7898, -15.7628) (-62.8684, -15.7322) (-62.9496, -15.7092) (-63.0327, -15.6944) (-63.1167, -15.687) (-63.201, -15.6864) (-63.2852, -15.6924) (-63.3687, -15.7042) (-63.4512, -15.7216) (-63.5325, -15.7436) (-63.6129, -15.769) (-63.7181, -15.8087) (-63.8458, -15.8672) (-63.9998, -15.9357) (-64.1563, -15.9983) (-64.3143, -16.0569) (-64.5269, -16.13) (-64.7955, -16.2125) (-65.1213, -16.2991) (-65.4499, -16.3745) (-65.7806, -16.4396) (-66.1132, -16.495) (-66.4471, -16.5414) (-66.7821, -16.579) (-67.1178, -16.6091) (-67.3422, -16.6224) (-67.4543, -16.6291) knots -1.078574 -1.078574 -1.078574 -1.078574 -1.044867 -1.011159 -0.977452 -0.943745 -0.910038 -0.876331 -0.842624 -0.808918 -0.775212 -0.758359 -0.741505 -0.724651 -0.707798 -0.690947 -0.68252 -0.674093 -0.665668 -0.657242 -0.648815 -0.640389 -0.631963 -0.623537 -0.61511 -0.606685 -0.598264 -0.589839 -0.581413 -0.57299 -0.564565 -0.556141 -0.539287 -0.522433 -0.514009 -0.505584 -0.49716 -0.488735 -0.48031 -0.471889 -0.463464 -0.455037 -0.446611 -0.438185 -0.429758 -0.421332 -0.412906 -0.40448 -0.396053 -0.387627 -0.370775 -0.353922 -0.337069 -0.320215 -0.303361 -0.269656 -0.235949 -0.202243 -0.168536 -0.134829 -0.101122 -0.067415 -0.033707 0 0 0 0 construction
  arc A22 (-68.1914, -15.3518) -> (-67.4543, -16.6291) centre (-40.1144, 0) ccw construction
  spline S19 degree 3 poles (-68.1914, -15.3518) (-68.1296, -15.258) (-68.0058, -15.0705) (-67.8117, -14.7948) (-67.6115, -14.5236) (-67.4043, -14.2577) (-67.1899, -13.9975) (-66.9681, -13.7437) (-66.7384, -13.4969) (-66.5004, -13.2581) (-66.2946, -13.0668) (-66.125, -12.9194) (-65.9952, -12.8119) (-65.8627, -12.7077) (-65.7263, -12.6086) (-65.6118, -12.5273) (-65.5247, -12.4561) (-65.4625, -12.3993) (-65.4028, -12.3398) (-65.3465, -12.277) (-65.2944, -12.2107) (-65.2472, -12.1408) (-65.2055, -12.0675) (-65.1698, -11.991) (-65.1411, -11.9117) (-65.1204, -11.8299) (-65.1076, -11.7465) (-65.1017, -11.6624) (-65.1061, -11.578) (-65.1185, -11.4946) (-65.1389, -11.4126) (-65.1803, -11.308) (-65.2401, -11.1809) (-65.2945, -11.0514) (-65.3445, -10.9506) (-65.3917, -10.8806) (-65.4454, -10.8156) (-65.5051, -10.7559) (-65.5716, -10.7039) (-65.6421, -10.6576) (-65.7167, -10.6182) (-65.7949, -10.5864) (-65.8755, -10.5617) (-65.9579, -10.5436) (-66.0415, -10.532) (-66.1256, -10.5262) (-66.2099, -10.526) (-66.2941, -10.5306) (-66.378, -10.5388) (-66.4891, -10.5558) (-66.6262, -10.5864) (-66.7911, -10.6214) (-66.9572, -10.6501) (-67.1239, -10.6746) (-67.347, -10.7018) (-67.6269, -10.7267) (-67.9636, -10.7437) (-68.3007, -10.7491) (-68.6377, -10.744) (-68.9745, -10.7291) (-69.3108, -10.705) (-69.6463, -10.6722) (-69.981, -10.6318) (-70.2032, -10.5982) (-70.3143, -10.5814) knots -1.078574 -1.078574 -1.078574 -1.078574 -1.044867 -1.011159 -0.977452 -0.943745 -0.910038 -0.876331 -0.842624 -0.808918 -0.775212 -0.758359 -0.741505 -0.724651 -0.707798 -0.690947 -0.68252 -0.674093 -0.665668 -0.657242 -0.648815 -0.640389 -0.631963 -0.623537 -0.61511 -0.606685 -0.598264 -0.589839 -0.581413 -0.57299 -0.564565 -0.556141 -0.539287 -0.522433 -0.514009 -0.505584 -0.49716 -0.488735 -0.48031 -0.471889 -0.463464 -0.455037 -0.446611 -0.438185 -0.429758 -0.421332 -0.412906 -0.40448 -0.396053 -0.387627 -0.370775 -0.353922 -0.337069 -0.320215 -0.303361 -0.269656 -0.235949 -0.202243 -0.168536 -0.134829 -0.101122 -0.067415 -0.033707 0 0 0 0 construction
  arc A23 (-70.7697, -9.1788) -> (-70.3143, -10.5814) centre (-40.1144, 0) ccw construction
  spline S20 degree 3 poles (-70.7697, -9.1788) (-70.6897, -9.0999) (-70.5296, -8.9422) (-70.2825, -8.7129) (-70.0303, -8.4892) (-69.7723, -8.2722) (-69.5085, -8.0623) (-69.2388, -7.8601) (-68.9628, -7.6665) (-68.6803, -7.4824) (-68.4392, -7.3381) (-68.2427, -7.2291) (-68.0934, -7.151) (-67.9421, -7.0766) (-67.7881, -7.0081) (-67.6592, -6.9523) (-67.5592, -6.9008) (-67.4866, -6.8581) (-67.4158, -6.8124) (-67.3476, -6.7627) (-67.2829, -6.7086) (-67.2222, -6.6501) (-67.1661, -6.5871) (-67.1154, -6.5197) (-67.0708, -6.448) (-67.0335, -6.3723) (-67.0037, -6.2935) (-66.9804, -6.2123) (-66.9672, -6.129) (-66.962, -6.0448) (-66.9649, -5.9604) (-66.9836, -5.8494) (-67.0157, -5.7127) (-67.0419, -5.5747) (-67.0699, -5.4657) (-67.1016, -5.3874) (-67.1405, -5.3126) (-67.1865, -5.2418) (-67.2407, -5.1771) (-67.3001, -5.1172) (-67.3649, -5.0632) (-67.4348, -5.0158) (-67.5085, -4.9749) (-67.5853, -4.9401) (-67.6646, -4.9113) (-67.7457, -4.8882) (-67.8281, -4.8704) (-67.9114, -4.8574) (-67.9952, -4.848) (-68.1074, -4.8415) (-68.2479, -4.843) (-68.4164, -4.8429) (-68.5849, -4.8364) (-68.7531, -4.8257) (-68.977, -4.806) (-69.2559, -4.7721) (-69.5888, -4.7188) (-69.9196, -4.654) (-70.2482, -4.5789) (-70.5746, -4.4943) (-70.8985, -4.4008) (-71.2198, -4.299) (-71.5388, -4.1899) (-71.7492, -4.1108) (-71.8543, -4.0713) knots -1.078574 -1.078574 -1.078574 -1.078574 -1.044867 -1.011159 -0.977452 -0.943745 -0.910038 -0.876331 -0.842624 -0.808918 -0.775212 -0.758359 -0.741505 -0.724651 -0.707798 -0.690947 -0.68252 -0.674093 -0.665668 -0.657242 -0.648815 -0.640389 -0.631963 -0.623537 -0.61511 -0.606685 -0.598264 -0.589839 -0.581413 -0.57299 -0.564565 -0.556141 -0.539287 -0.522433 -0.514009 -0.505584 -0.49716 -0.488735 -0.48031 -0.471889 -0.463464 -0.455037 -0.446611 -0.438185 -0.429758 -0.421332 -0.412906 -0.40448 -0.396053 -0.387627 -0.370775 -0.353922 -0.337069 -0.320215 -0.303361 -0.269656 -0.235949 -0.202243 -0.168536 -0.134829 -0.101122 -0.067415 -0.033707 0 0 0 0 construction
  arc A24 (-72.0082, -2.6046) -> (-71.8543, -4.0713) centre (-40.1144, 0) ccw construction
  spline S21 degree 3 poles (-72.0082, -2.6046) (-71.9135, -2.5441) (-71.7242, -2.4231) (-71.4348, -2.2502) (-71.1416, -2.0839) (-70.8441, -1.9252) (-70.5424, -1.7747) (-70.2365, -1.6331) (-69.9263, -1.501) (-69.6118, -1.3797) (-69.346, -1.2887) (-69.1311, -1.2229) (-68.9687, -1.1776) (-68.8053, -1.1363) (-68.6404, -1.1013) (-68.5027, -1.0735) (-68.3943, -1.0439) (-68.3143, -1.0173) (-68.2355, -0.9873) (-68.1586, -0.9528) (-68.084, -0.9134) (-68.0125, -0.8688) (-67.9445, -0.8188) (-67.8809, -0.7634) (-67.8224, -0.7026) (-67.7702, -0.6363) (-67.7246, -0.5653) (-67.685, -0.4908) (-67.6546, -0.412) (-67.6321, -0.3307) (-67.6173, -0.2476) (-67.6126, -0.1352) (-67.6156, 0.0053) (-67.6126, 0.1457) (-67.6172, 0.2581) (-67.6319, 0.3413) (-67.6545, 0.4225) (-67.6848, 0.5014) (-67.7243, 0.5759) (-67.7699, 0.6468) (-67.8221, 0.7132) (-67.8806, 0.774) (-67.9442, 0.8294) (-68.0121, 0.8794) (-68.0837, 0.9241) (-68.1582, 0.9635) (-68.2352, 0.998) (-68.3139, 1.028) (-68.3939, 1.0547) (-68.5023, 1.0844) (-68.64, 1.1122) (-68.8049, 1.1473) (-68.9683, 1.1886) (-69.1306, 1.234) (-69.3455, 1.2999) (-69.6112, 1.391) (-69.9258, 1.5124) (-70.2359, 1.6446) (-70.5418, 1.7864) (-70.8433, 1.937) (-71.1408, 2.0957) (-71.4339, 2.2622) (-71.7232, 2.4352) (-71.9125, 2.5563) (-72.0072, 2.6168) knots -1.078574 -1.078574 -1.078574 -1.078574 -1.044867 -1.011159 -0.977452 -0.943745 -0.910038 -0.876331 -0.842624 -0.808918 -0.775212 -0.758359 -0.741505 -0.724651 -0.707798 -0.690947 -0.68252 -0.674093 -0.665668 -0.657242 -0.648815 -0.640389 -0.631963 -0.623537 -0.61511 -0.606685 -0.598264 -0.589839 -0.581413 -0.57299 -0.564565 -0.556141 -0.539287 -0.522433 -0.514009 -0.505584 -0.49716 -0.488735 -0.48031 -0.471889 -0.463464 -0.455037 -0.446611 -0.438185 -0.429758 -0.421332 -0.412906 -0.40448 -0.396053 -0.387627 -0.370775 -0.353922 -0.337069 -0.320215 -0.303361 -0.269656 -0.235949 -0.202243 -0.168536 -0.134829 -0.101122 -0.067415 -0.033707 0 0 0 0 construction
  arc A25 (-71.8528, 4.0834) -> (-72.0072, 2.6168) centre (-40.1144, 0) ccw construction
  spline S22 degree 3 poles (-71.8528, 4.0834) (-71.7476, 4.1229) (-71.5372, 4.2019) (-71.2182, 4.3109) (-70.8968, 4.4126) (-70.5728, 4.5059) (-70.2465, 4.5904) (-69.9178, 4.6654) (-69.5869, 4.73) (-69.254, 4.7833) (-68.9751, 4.817) (-68.7512, 4.8367) (-68.583, 4.8473) (-68.4146, 4.8537) (-68.246, 4.8537) (-68.1056, 4.8522) (-67.9933, 4.8586) (-67.9096, 4.8681) (-67.8263, 4.881) (-67.7438, 4.8987) (-67.6627, 4.9218) (-67.5834, 4.9506) (-67.5066, 4.9853) (-67.4328, 5.0263) (-67.363, 5.0736) (-67.2981, 5.1276) (-67.2388, 5.1875) (-67.1845, 5.2522) (-67.1385, 5.3229) (-67.0995, 5.3977) (-67.0678, 5.476) (-67.0398, 5.585) (-67.0135, 5.723) (-66.9814, 5.8597) (-66.9626, 5.9706) (-66.9597, 6.055) (-66.9648, 6.1392) (-66.9781, 6.2226) (-67.0013, 6.3037) (-67.0311, 6.3826) (-67.0683, 6.4584) (-67.1129, 6.53) (-67.1636, 6.5974) (-67.2197, 6.6605) (-67.2804, 6.719) (-67.3451, 6.7731) (-67.4131, 6.8228) (-67.4839, 6.8686) (-67.5566, 6.9113) (-67.6565, 6.9629) (-67.7854, 7.0187) (-67.9394, 7.0873) (-68.0906, 7.1617) (-68.2399, 7.2399) (-68.4364, 7.349) (-68.6775, 7.4933) (-68.9599, 7.6775) (-69.2358, 7.8712) (-69.5054, 8.0735) (-69.7691, 8.2836) (-70.027, 8.5007) (-70.2792, 8.7244) (-70.5262, 8.9538) (-70.6862, 9.1116) (-70.7662, 9.1905) knots -1.078574 -1.078574 -1.078574 -1.078574 -1.044867 -1.011159 -0.977452 -0.943745 -0.910038 -0.876331 -0.842624 -0.808918 -0.775212 -0.758359 -0.741505 -0.724651 -0.707798 -0.690947 -0.68252 -0.674093 -0.665668 -0.657242 -0.648815 -0.640389 -0.631963 -0.623537 -0.61511 -0.606685 -0.598264 -0.589839 -0.581413 -0.57299 -0.564565 -0.556141 -0.539287 -0.522433 -0.514009 -0.505584 -0.49716 -0.488735 -0.48031 -0.471889 -0.463464 -0.455037 -0.446611 -0.438185 -0.429758 -0.421332 -0.412906 -0.40448 -0.396053 -0.387627 -0.370775 -0.353922 -0.337069 -0.320215 -0.303361 -0.269656 -0.235949 -0.202243 -0.168536 -0.134829 -0.101122 -0.067415 -0.033707 0 0 0 0 construction
  arc A26 (-70.3102, 10.593) -> (-70.7662, 9.1905) centre (-40.1144, 0) ccw construction